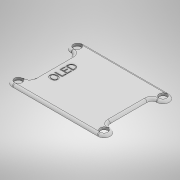
# Autodesk Inventor part: OledModCover
Saved by Autodesk Inventor 2021 (Build 250183000, 183)
## iProperties
Created: 2021-08-19
Part Number: OledModCover
Material: Generic
Document SubType Name: Modeling
Designer: perez
Density: 1 g/cm^3
Appearance: Default
Author: perez
Autodesk Inventor part; units mm, degrees
ref_plane "YZ Plane" through (0, 0, 0) normal (1, 0, 0) x (0, 1, 0)
ref_plane "XZ Plane" through (0, 0, 0) normal (0, 1, 0) x (-1, 0, 0)
ref_plane "XY Plane" through (0, 0, 0) normal (0, 0, 1) x (1, 0, 0)
sketch "Sketch1" plane through (0, 0, 0) normal (0, 1, 0) x (-1, 0, 0)
  line L0 (0, 0) -> (27, 0) construction
  line L1 (27, -25) -> (0, -25) construction
  line L2 (0, -25) -> (0, 0) construction
  line L3 (31, 2) -> (-4, 2)
  line L4 (-4, -27) -> (31, -27)
  line L5 (29, -22) -> (29, -3)
  arc A0 (31, -3) -> (31, 2) centre (31, -0.5) ccw
  arc A1 (31, -27) -> (31, -22) centre (31, -24.5) ccw
  arc A2 (-4, 2) -> (-4, -3) centre (-4, -0.5) ccw
  arc A3 (-4, -22) -> (-4, -27) centre (-4, -24.5) ccw
  line L6 (31, -3) -> (29, -3)
  line L7 (31, -22) -> (29, -22)
  line L8 (-4, -3) -> (-2, -3)
  line L9 (-4, -22) -> (-2, -22)
  line L10 (-2, -3) -> (-2, -22)
  circle A4 centre (31, -0.5) radius 1.55
  circle A5 centre (31, -24.5) radius 1.55
  circle A6 centre (-4, -0.5) radius 1.55
  circle A7 centre (-4, -24.5) radius 1.55
  line L11 (21.5, -25) -> (7.5, -25)
  line L12 (7.5, -25) -> (7.5, 0)
  line L13 (7.5, 0) -> (21.5, 0)
  line L14 (21.5, 0) -> (21.5, -25)
  point P0 (29, 2)
  point P1 (-2, -27)
  point P2 (-2, 2)
  point P3 (29, -27)
  dimension "d0" = 27
  dimension "d1" = 25
  dimension "d12" = 2
  dimension "d14" = 2
  dimension "d22" = 5
  dimension "d23" = 2.5
  dimension "d24" = 2
  dimension "d25" = 2.5
  dimension "d26" = 2
  dimension "d27" = 5
  dimension "d28" = 5
  dimension "d29" = 5
  dimension "d32" = 2.5
  dimension "d33" = 2.5
  dimension "d34" = 3.1
  dimension "d35" = 3.1
  dimension "d36" = 3.1
  dimension "d37" = 3.1
  dimension "d47" = 2
  dimension "d48" = 2
  dimension "d49" = 7.5
  dimension "d50" = 14
  constraints: 30 end point, 8 centre point, 8 point on circle, 6 parallel, 6 point on line, 4 coincident, 4 perpendicular, 3 horizontal, 3 tangent
  measures "d0" distance of L1.start L1.end
  measures "d1" distance of L0.end L1.start
  measures "d12" distance between parallel lines of L4 L1
  measures "d14" distance between parallel lines of L0 L3
  measures "d22" diameter of A0
  measures "d23" distance from line of L3 A0.centre
  measures "d24" distance from line of L5 A0.centre
  measures "d25" distance from line of L4 A1.centre
  measures "d26" distance from line of L5 A1.centre
  measures "d27" diameter of A1
  measures "d28" diameter of A2
  measures "d29" diameter of A3
  measures "d32" distance from line of L4 A3.centre
  measures "d33" distance from line of L3 A2.centre
  measures "d34" diameter of A4
  measures "d35" diameter of A5
  measures "d36" diameter of A6
  measures "d37" diameter of A7
  measures "d47" distance between parallel lines of L11 L4
  measures "d48" distance between parallel lines of L3 L13
  measures "d49" distance between parallel lines of L2 L12
  measures "d50" distance between parallel lines of L12 L14
extrude "Extrusion1" add sketch "Sketch1" against normal blind 1 contours A0 L6 L5 L7 A1 L4 A3 L9 L10 L8 A2 L3 | L11 L12 L13 L14
fillet "Fillet2" radius 2 4 edges at (2, -0.5, -22) (2, -0.5, -3) (-29, -0.5, -3) (-29, -0.5, -22)
fillet "Fillet3" radius 1 12 edges at (6.5, 0, -0.5) (4, 0, -3) (2, 0, -12.5) (3.9999, 0, -22) (6.5, 0, -24.5) (-13.5, 0, -27) (-33.5, 0, -24.5) (-31, 0, -22) (-29, 0, -12.5) (-31, 0, -3) (-33.5, 0, -0.5) (-13.5, 0, 2)
sketch "Sketch4" plane through (0, 0, 0) normal (0, 1, 0) x (1, 0, 0)
  line L0 (-26.4552, 7.4269) -> (-26.4552, 17.6726) construction
  line L1 (-26.4552, 17.6726) -> (-23.2788, 17.6726) construction
  line L2 (-23.2788, 17.6726) -> (-23.2788, 7.4269) construction
  line L3 (-23.2788, 7.4269) -> (-26.4552, 7.4269) construction
  spline S0 degree 2 poles (-26.0427, 9.892) (-25.8402, 10.0649) (-25.2474, 10.2576) (-24.867, 10.2576) knots 0 0 0 1 2 2 2
  spline S1 degree 2 poles (-24.867, 10.2576) (-24.4965, 10.2576) (-23.8963, 10.0698) (-23.6937, 9.892) knots 0 0 0 1 2 2 2
  spline S2 degree 2 poles (-23.6937, 9.892) (-23.4813, 9.7043) (-23.2788, 9.2078) (-23.2788, 8.9089) knots 0 0 0 1 2 2 2
  spline S3 degree 2 poles (-23.2788, 8.9089) (-23.2788, 8.6002) (-23.4887, 8.1062) (-23.6937, 7.9259) knots 0 0 0 1 2 2 2
  spline S4 degree 2 poles (-23.6937, 7.9259) (-23.8963, 7.7505) (-24.4915, 7.5628) (-24.867, 7.5628) knots 0 0 0 1 2 2 2
  spline S5 degree 2 poles (-24.867, 7.5628) (-25.2498, 7.5628) (-25.8328, 7.753) (-26.0427, 7.9283) knots 0 0 0 1 2 2 2
  spline S6 degree 2 poles (-26.0427, 7.9283) (-26.2453, 8.1062) (-26.4552, 8.6027) (-26.4552, 8.9089) knots 0 0 0 1 2 2 2
  spline S7 degree 2 poles (-26.4552, 8.9089) (-26.4552, 9.2202) (-26.2378, 9.7191) (-26.0427, 9.892) knots 0 0 0 1 2 2 2
  spline S8 degree 2 poles (-24.867, 9.8352) (-25.1683, 9.8352) (-25.6352, 9.7043) (-25.7883, 9.5857) knots 0 0 0 1 2 2 2
  spline S9 degree 2 poles (-25.7883, 9.5857) (-25.9464, 9.4647) (-26.1045, 9.1238) (-26.1045, 8.9114) knots 0 0 0 1 2 2 2
  spline S10 degree 2 poles (-26.1045, 8.9114) (-26.1045, 8.6916) (-25.9513, 8.3606) (-25.7883, 8.2346) knots 0 0 0 1 2 2 2
  spline S11 degree 2 poles (-25.7883, 8.2346) (-25.6327, 8.1136) (-25.1634, 7.9851) (-24.867, 7.9851) knots 0 0 0 1 2 2 2
  spline S12 degree 2 poles (-24.867, 7.9851) (-24.2668, 7.9851) (-23.6295, 8.489) (-23.6295, 8.9114) knots 0 0 0 1 2 2 2
  spline S13 degree 2 poles (-23.6295, 8.9114) (-23.6295, 9.3338) (-24.2668, 9.8352) (-24.867, 9.8352) knots 0 0 0 1 2 2 2
  line L4 (-23.343, 12.4682) -> (-23.343, 10.7022)
  line L5 (-23.343, 10.7022) -> (-26.391, 10.7022)
  line L6 (-26.391, 10.7022) -> (-26.391, 11.1073)
  line L7 (-26.391, 11.1073) -> (-23.7036, 11.1073)
  line L8 (-23.7036, 11.1073) -> (-23.7036, 12.4682)
  line L9 (-23.7036, 12.4682) -> (-23.343, 12.4682)
  line L10 (-23.343, 12.7869) -> (-26.391, 12.7869)
  line L11 (-26.391, 12.7869) -> (-26.391, 14.6937)
  line L12 (-26.391, 14.6937) -> (-26.0304, 14.6937)
  line L13 (-26.0304, 14.6937) -> (-26.0304, 13.1919)
  line L14 (-26.0304, 13.1919) -> (-25.1955, 13.1919)
  line L15 (-25.1955, 13.1919) -> (-25.1955, 14.5924)
  line L16 (-25.1955, 14.5924) -> (-24.8349, 14.5924)
  line L17 (-24.8349, 14.5924) -> (-24.8349, 13.1919)
  line L18 (-24.8349, 13.1919) -> (-23.7036, 13.1919)
  line L19 (-23.7036, 13.1919) -> (-23.7036, 14.6937)
  line L20 (-23.7036, 14.6937) -> (-23.343, 14.6937)
  line L21 (-23.343, 14.6937) -> (-23.343, 12.7869)
  spline S14 degree 2 poles (-24.8645, 17.5416) (-24.4471, 17.5416) (-23.7752, 17.2033) (-23.5875, 16.9192) knots 0 0 0 1 2 2 2
  spline S15 degree 2 poles (-23.5875, 16.9192) (-23.4418, 16.687) (-23.343, 16.2103) (-23.343, 15.8398) knots 0 0 0 1 2 2 2
  line L22 (-23.343, 15.8398) -> (-23.343, 15.1383)
  line L23 (-23.343, 15.1383) -> (-26.391, 15.1383)
  line L24 (-26.391, 15.1383) -> (-26.391, 15.8324)
  spline S16 degree 2 poles (-26.391, 15.8324) (-26.391, 16.2622) (-26.2625, 16.7512) (-26.1489, 16.9241) knots 0 0 0 1 2 2 2
  spline S17 degree 2 poles (-26.1489, 16.9241) (-25.9538, 17.2181) (-25.3091, 17.5416) (-24.8645, 17.5416) knots 0 0 0 1 2 2 2
  spline S18 degree 2 poles (-24.8695, 17.1193) (-25.2202, 17.1193) (-25.7167, 16.8871) (-25.8575, 16.6574) knots 0 0 0 1 2 2 2
  spline S19 degree 2 poles (-25.8575, 16.6574) (-25.9538, 16.4944) (-26.0402, 16.1263) (-26.0402, 15.8522) knots 0 0 0 1 2 2 2
  line L25 (-26.0402, 15.8522) -> (-26.0402, 15.5434)
  line L26 (-26.0402, 15.5434) -> (-23.6937, 15.5434)
  line L27 (-23.6937, 15.5434) -> (-23.6937, 15.8522)
  spline S20 degree 2 poles (-23.6937, 15.8522) (-23.6937, 16.1214) (-23.7802, 16.5289) (-23.8963, 16.6944) knots 0 0 0 1 2 2 2
  spline S21 degree 2 poles (-23.8963, 16.6944) (-24.0395, 16.9068) (-24.5138, 17.1193) (-24.8695, 17.1193) knots 0 0 0 1 2 2 2
  point P0 (0, 0)
  constraints: 2 other
emboss "Emboss2" sketch "Sketch4" operation cut depth 0.2 direction (0, -1, 0)
sketch "Sketch5" plane through (0, 0, 0) normal (0, 1, 0) x (1, 0, 0)
  line L0 (-36.8422, 31.8263) -> (7.3356, 31.8263)
  line L1 (7.3356, 31.8263) -> (7.3356, 26.5)
  line L2 (7.3356, 26.5) -> (-36.8422, 26.5)
  line L3 (-36.8422, 26.5) -> (-36.8422, 31.8263)
  line L4 (-30.6095, 27) -> (3.6095, 27) projected
  point P0 (0, 0)
  dimension "d58" = 0.5
  constraints: 8 end point, 2 parallel, 1 horizontal, 1 perpendicular
  measures "d58" distance between parallel lines of L2 L4
extrude "Extrusion3" cut sketch "Sketch5" against normal blind 10
equation "\"d14\" = d12"
equation "\"d15\" = d12"
body "Solid1"
